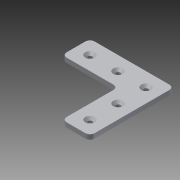
# Autodesk Inventor part: angle-90-plate
Saved by Autodesk Inventor 2013 (Build 170138000, 138)
## iProperties
Created: 2013-09-15
Part Number: angle-90-plate
Material: Aluminum 6061
Document SubType Name: Modeling
Designer: Ian
Density: 2.71 g/cm^3
Mass: 119.202 g
Surface Area: 174.354 cm^2
Volume: 43.986 cm^3
Author: Ian
Autodesk Inventor part; units mm, degrees
ref_plane "YZ Plane" through (0, 0, 0) normal (1, 0, 0) x (0, 1, 0)
ref_plane "XZ Plane" through (0, 0, 0) normal (0, 1, 0) x (-1, 0, 0)
ref_plane "XY Plane" through (0, 0, 0) normal (0, 0, 1) x (1, 0, 0)
sketch "Sketch1" plane through (0, 0, 0) normal (0, 1, 0) x (-1, 0, 0)
  line L0 (0, 0) -> (19.05, 0)
  line L1 (38.1, 38.1) -> (38.1, 114.3)
  line L2 (38.1, 114.3) -> (0, 114.3)
  line L3 (0, 114.3) -> (0, 0)
  line L4 (0, 0) -> (114.3, 0)
  line L5 (114.3, 0) -> (114.3, 38.1)
  line L6 (114.3, 38.1) -> (38.1, 38.1)
  line L7 (0, 38.1) -> (0, 0)
  line L8 (19.05, 114.3) -> (19.05, 19.05) construction
  line L9 (19.05, 19.05) -> (114.3, 19.05) construction
  point P0 (19.05, 95.25)
  point P1 (19.05, 57.15)
  point P2 (57.15, 19.05)
  point P3 (95.25, 19.05)
  dimension "d3" = 38.1
  dimension "d4" = 114.3
  dimension "d5" = 114.3
  dimension "d6" = 38.1
  dimension "d9" = 19.05
  dimension "d10" = 19.05
  dimension "d11" = 19.05
  dimension "d12" = 57.15
  dimension "d13" = 19.05
  dimension "d14" = 57.15
  constraints: 20 end point, 5 parallel, 5 point on line, 3 perpendicular, 2 horizontal, 2 midpoint, 1 coincident
  measures "d3" distance of L5.end L4.end
  measures "d4" distance of L0.start L4.end
  measures "d5" distance of L2.end L0.start
  measures "d6" distance of L1.end L2.end
  measures "d9" distance from line of L4.end L9
  measures "d10" distance from line of L8 L2.end
  measures "d11" distance from line of L5 point (95.25, 19.05)
  measures "d12" distance from line of point (57.15, 19.05) L5
  measures "d13" distance from line of point (19.05, 95.25) L2
  measures "d14" vertical distance of point (19.05, 57.15) L2.end
extrude "Extrusion1" add sketch "Sketch1" against normal blind 6.35
hole "Hole1" at (-19.05, 0, 95.25) at (-19.05, 0, 57.15) at (-57.15, 0, 19.05) at (-95.25, 0, 19.05) at (-19.05, 0, 19.05) direction (0, -1, 0) diameter 6.7564 end through all countersink diameter 12.8778 countersink angle 82 clearance for "Flat Head Machine Screw (82)" size "1/4" standard "Ansi Unified Screw Threads"
fillet "Fillet1" radius 6.35 6 edges at (0, -3.175, 114.3) (0, -3.175, 0) (-38.1, -3.175, 114.3) (-38.1, -3.175, 38.1) (-114.3, -3.175, 0) (-114.3, -3.175, 38.1)
equation "\"d3\" = d6"
equation "\"d4\" = d5"
equation "\"d9\" = d10"
equation "\"d11\" = d13"
equation "\"d12\" = d14"
body "Solid1"
